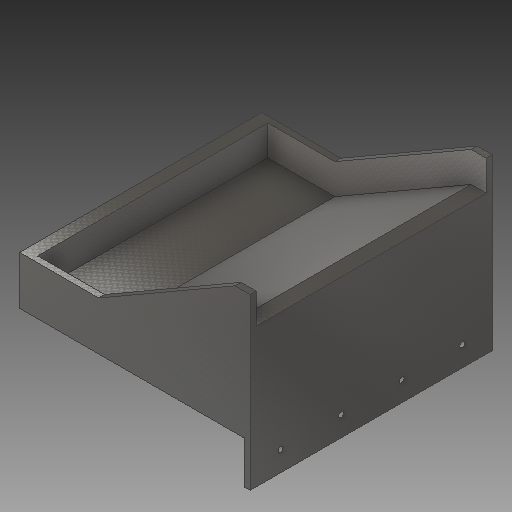
# Autodesk Inventor part: rampa
Saved by Autodesk Inventor 2019 (Build 230136000, 136)
## iProperties
Created: 2019-02-26
Part Number: rampa
Material: Generic
Document SubType Name: Modeling
Designer: felix
Density: 1 g/cm^3
Appearance: Default
Mass: 12760.4 g
Surface Area: 6251.95 cm^2
Volume: 12760.4 cm^3
Author: felix
Autodesk Inventor part; units mm, degrees
ref_plane "YZ Plane" through (0, 0, 0) normal (1, 0, 0) x (0, 1, 0)
ref_plane "XZ Plane" through (0, 0, 0) normal (0, 1, 0) x (-1, 0, 0)
sketch "Sketch1" plane through (0, 0, 0) normal (0, 0, 1) x (1, 0, 0)
  line L0 (0, 0) -> (225.1666, 130)
  line L1 (0, 0) -> (260, 0) construction
  line L2 (225.1666, 130) -> (250.1666, 130)
  line L3 (250.1666, 130) -> (250.1666, 0)
  line L4 (250.1666, 0) -> (0, 0)
  dimension "d4" = 30
  dimension "d5" = 260
  dimension "d6" = 25
  constraints: 10 end point, 2 horizontal, 2 perpendicular, 1 equal length
  measures "d4" angle of L1 L0
  measures "d5" distance of L0.start L0.end
  measures "d6" distance of L0.end L2.end
extrude "Extrusion1" add sketch "Sketch1" along normal blind 200 and the other way blind 200
sketch "Sketch8" plane through (250.1666, 0, -200) normal (0, -1, 0) x (1, 0, 0)
  line L0 (0, 0) -> (-250.1666, 0) projected
  line L1 (0, 400) -> (0, 390) projected
  line L2 (-260.64, 0) -> (0, 0)
  line L3 (0, 0) -> (0, 400)
  line L4 (0, 400) -> (-260.64, 400)
  line L5 (-260.64, 400) -> (-260.64, 0)
  point P0 (-250.1666, 200)
  constraints: 8 end point, 2 parallel, 1 horizontal, 1 perpendicular
extrude "Extrusion8" add sketch "Sketch8" along normal blind 30
sketch "Sketch9" plane through (-10.4734, -30, -200) normal (-1, 0, 0) x (0, 0, 1)
  line L0 (0, 160) -> (0, 0) projected
  line L1 (400, 160) -> (400, 0) projected
  line L2 (0, 0) -> (400, 0)
  line L3 (400, 0) -> (400, 30)
  line L4 (400, 30) -> (0, 30)
  line L5 (0, 30) -> (0, 0)
  point P0 (200, 30)
  point P1 (0, 229.8807)
  point P2 (400, 229.8807)
  constraints: 8 end point, 2 parallel, 1 horizontal, 1 perpendicular, 1 point on line
extrude "Extrusion9" add sketch "Sketch9" along normal blind 120
sketch "Sketch10" plane through (-130.4734, 0, -200) normal (0, 1, 0) x (1, 0, 0)
  line L0 (380.64, -400) -> (0, -400) projected
  line L1 (380.64, 0) -> (0, 0) projected
  line L2 (0, -400) -> (20, -400)
  line L3 (20, -400) -> (20, 0)
  line L4 (20, 0) -> (0, 0)
  line L5 (0, 0) -> (0, -400)
  point P0 (130.4734, -200)
  dimension "d32" = 20
  constraints: 8 end point, 2 parallel, 1 horizontal, 1 perpendicular, 1 point on line
  measures "d32" distance between parallel lines of L5 L3
extrude "Extrusion10" add sketch "Sketch10" along normal blind 50
sketch "Sketch11" plane through (0, 0, -200) normal (0, 0, -1) x (-1, 0, 0)
  line L0 (-250.1666, 130) -> (-250.1666, -30) projected
  line L1 (-250.1666, 130) -> (-250.1666, 180)
  line L2 (0, 0) -> (-225.1666, 130) projected
  line L3 (0, 0) -> (0, 50)
  line L4 (110.4734, 0) -> (110.4734, 50) projected
  line L5 (0, 50) -> (110.4734, 50)
  line L6 (0, 50) -> (-225.1666, 180)
  line L7 (-225.1666, 180) -> (-250.1666, 180)
  line L8 (-225.1666, 130) -> (-225.1666, 180)
  line L9 (-225.1666, 130) -> (-250.1666, 130) projected
  line L10 (0, 0) -> (110.4734, 0) projected
  dimension "d35" = 50
  dimension "d36" = 50
  constraints: 12 end point, 2 vertical, 1 horizontal, 1 perpendicular
  measures "d35" distance of L0.start L1.end
  measures "d36" distance of L2.start L3.end
extrude "Extrusion11" add sketch "Sketch11" against normal blind 10
ref_plane "Work Plane2" through (250.1666, 130, 0) normal (0, 0, -1) x (-1, 0, 0)
ref_plane "Work Plane1" through (250.1666, 130, 5) normal (0, 0, -1) x (-1, 0, 0)
mirror "Mirror1" about plane through (250.1666, 130, 0) normal (0, 0, -1) of "Extrusion11"
sketch "Sketch12" plane through (250.1666, -30, -200) normal (0, -1, 0) x (1, 0, 0)
  line L0 (0, 400) -> (-380.64, 400) projected
  line L1 (0, 400) -> (-10, 400)
  line L2 (-10, 400) -> (-10, 0)
  line L3 (-10, 0) -> (0, 0)
  line L4 (0, 0) -> (0, 400)
  point P0 (-250.1666, 200)
  dimension "d40" = 10
  constraints: 8 end point, 2 parallel, 1 horizontal, 1 perpendicular
  measures "d40" distance of L3.end L2.end
extrude "Extrusion12" add sketch "Sketch12" along normal blind 70
sketch "Sketch13" plane through (240.1666, -30, -200) normal (-1, 0, 0) x (0, 0, 1)
  line L0 (0, 0) -> (0, -70) projected
  line L1 (0, 0) -> (400, 0) projected
  point P0 (200, 30)
  point P1 (50, -37)
  dimension "d43" = 50
  dimension "d44" = 37
  measures "d43" distance from line of L0 point (50, -37)
  measures "d44" distance from line of L1 point (50, -37)
hole "Hole1" at (240.1666, -67, -150) direction (1, 0, 0) diameter 8.376 depth 27.3 tip angle 118 thread size "M10x1.5" class "6H" standard "ISO Metric profile"
pattern_linear "Rectangular Pattern1" count 4 spacing 100 along (0, 0, 1) of "Hole1"
body "Solid1"
